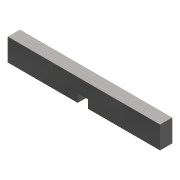
# Autodesk Inventor part: Slide_Key
Saved by Autodesk Inventor 2022 (Build 260148000, 148)
## iProperties
Created: 2006-01-18
Part Number: Slide_Key
Document SubType Name: Modeling
Designer: PMiller
Material: Steel, High Strength Low Alloy
Density: 7.84 g/cm^3
Appearance: Steel - Polished
Author: PMiller
Autodesk Inventor part; units mm, degrees
ref_plane "YZ Plane" through (0, 0, 0) normal (1, 0, 0) x (0, 1, 0)
ref_plane "XZ Plane" through (0, 0, 0) normal (0, 1, 0) x (-1, 0, 0)
sketch "Sketch1" plane through (0, 0, 0) normal (0, 0, 1) x (1, 0, 0)
  line L0 (-29.3688, -4.318) -> (-29.3688, 4.318)
  line L1 (-29.3688, 4.318) -> (29.3688, 4.318)
  line L2 (29.3688, 4.318) -> (29.3688, -4.318)
  line L3 (29.3688, -4.318) -> (1.5875, -4.318)
  line L4 (1.5875, -4.318) -> (1.5875, -1.143)
  line L5 (1.5875, -1.143) -> (-2.3812, -1.143)
  line L6 (-2.3812, -1.143) -> (-2.3812, -4.318)
  line L7 (-2.3812, -4.318) -> (-29.3688, -4.318)
  point P0 (0, 0)
  point P1 (0, 4.318)
  point P2 (-29.3688, 0)
  dimension "d0" = 58.7375
  dimension "d1" = 3.9688
  dimension "d2" = 3.175
  dimension "d3" = 27.7812
  dimension "d4" = 8.636
  constraints: 16 end point, 7 parallel, 2 midpoint, 1 horizontal alignment, 1 perpendicular, 1 vertical, 1 vertical alignment
  measures "d0" distance of L0.end L1.end
  measures "d1" distance of L4.end L5.end
  measures "d2" distance of L3.end L4.end
  measures "d3" distance between parallel lines of L2 L4
  measures "d4" distance of L1.end L2.end
extrude "Extrusion1" add sketch "Sketch1" along normal mid plane 4.699
ref_plane "Work Plane1" through (-0.3969, -4.318, 2.3495) normal (1, 0, 0) x (0, 0, -1)
body "Solid1"
